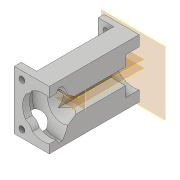
# Autodesk Inventor part: 30_CUBE_OpenSIM_Beamexpander
Saved by Autodesk Inventor 2019 (Build 230136000, 136)
## iProperties
Created: 2019-10-21
Part Number: 30_CUBE_OpenSIM_Beamexpander
Material: Generic
Document SubType Name: Modeling
Designer: diederichbenedict
Density: 1 g/cm^3
Appearance: Default
Author: diederichbenedict
Autodesk Inventor part; units mm, degrees
ref_plane "YZ Plane" through (0, 0, 0) normal (1, 0, 0) x (0, 1, 0)
ref_plane "XZ Plane" through (0, 0, 0) normal (0, 1, 0) x (-1, 0, 0)
ref_plane "XY Plane" through (0, 0, 0) normal (0, 0, 1) x (1, 0, 0)
ref_plane "Work Plane1" through (0, 0, 0) normal (0, 0, 1) x (1, 0, 0)
sketch "Sketch1" plane through (0, 0, 0) normal (0, 0, 1) x (1, 0, 0)
  circle A0 centre (11, -11) radius 1 projected
  circle A1 centre (-11, -11) radius 1 projected
  circle A2 centre (-11, 11) radius 1 projected
  circle A3 centre (11, 11) radius 1 projected
  circle A4 centre (0, 0) radius 2.8472 projected
  circle A5 centre (0, 0) radius 9.9557 construction
  line L0 (12.95, 14.95) -> (-12.95, 14.95) construction
  arc A6 (-12.95, 14.95) -> (-14.95, 12.95) centre (-12.95, 12.95) ccw construction
  line L1 (-14.95, 12.95) -> (-14.95, -12.95) construction
  arc A7 (-14.95, -12.95) -> (-12.95, -14.95) centre (-12.95, -12.95) ccw construction
  line L2 (-12.95, -14.95) -> (12.95, -14.95) construction
  arc A8 (12.95, -14.95) -> (14.95, -12.95) centre (12.95, -12.95) ccw construction
  line L3 (14.95, -12.95) -> (14.95, 12.95) construction
  arc A9 (14.95, 12.95) -> (12.95, 14.95) centre (12.95, 12.95) ccw construction
  line L4 (-14.95, -14.95) -> (10.05, -14.95) construction
  line L5 (10.05, -14.95) -> (10.05, 14.95) construction
  line L6 (10.05, 14.95) -> (-14.95, 14.95) construction
  line L7 (-14.95, 14.95) -> (-14.95, -14.95) construction
  line L8 (-14.95, -14.95) -> (10.05, -14.95)
  line L9 (10.05, -14.95) -> (10.05, 14.95)
  line L10 (10.05, 14.95) -> (-14.95, 14.95)
  line L11 (-14.95, 14.95) -> (-14.95, -14.95)
  circle A10 centre (-11, -11) radius 1.5
  circle A11 centre (-11, 11) radius 1.5
  line L12 (2.9776, -9.5) -> (2.9776, -14.95)
  line L13 (2.9776, 9.5) -> (2.9776, 14.95)
  arc A12 (2.9776, 9.5) -> (2.9776, -9.5) centre (0, 0) ccw
  point P0 (0, 0)
  dimension "d0" = 25
  dimension "d1" = 3
  dimension "d2" = 3
  constraints: 20 end point, 5 point on line, 4 parallel, 4 point on circle, 3 centre point, 3 perpendicular, 2 coincident, 2 horizontal, 1 concentric
  measures "d0" distance of L6.end L5.end
  measures "d1" diameter of A10
  measures "d2" diameter of A11
extrude "Extrusion1" add sketch "Sketch1" along normal blind 3 contours L8 L11 L10 L13 A12 L12
sketch "Sketch2" plane through (0, 0, 3) normal (0, 0, 1) x (1, 0, 0)
  circle A0 centre (-11, 11) radius 1.5 projected
  circle A1 centre (-11, -11) radius 1.5 projected
  line L0 (-14.95, -14.95) -> (2.9776, -14.95) projected
  line L1 (2.9776, -14.95) -> (2.9776, -9.5) projected
  arc A2 (2.9776, 9.5) -> (2.9776, -9.5) centre (0, 0) ccw projected
  line L2 (2.9776, 9.5) -> (2.9776, 14.95) projected
  line L3 (2.9776, 14.95) -> (-14.95, 14.95) projected
  line L4 (-14.95, 14.95) -> (-14.95, -14.95) projected
  line L5 (2.9776, -9.5) -> (2.9776, 9.5)
  circle A3 centre (-11, -11) radius 1.5 projected
  line L6 (-14.95, -14.95) -> (2.9776, -14.95) projected
  circle A4 centre (-11, -11) radius 5.5861
  line L7 (2.9776, 14.95) -> (-14.95, 14.95) projected
  circle A5 centre (-11, 11) radius 5.5861
  arc A6 (2.9776, 9.5) -> (2.9776, -9.5) centre (0, 0) ccw projected
  circle A7 centre (0, 0) radius 2.9776
  line L8 (0, -2.9776) -> (2.9776, -2.9776)
  line L9 (0, 2.9776) -> (2.9776, 2.9776)
  point P0 (0, 0)
  point P1 (-14.95, -7.05)
  point P2 (-7.0295, -7.05)
  point P3 (-7.05, -14.95)
  point P4 (-7.05, 7.05)
  point P5 (-14.95, 7.05)
  point P6 (-7.05, 14.95)
  constraints: 10 point on circle, 6 end point, 6 point on line, 3 centre point, 3 coincident, 2 perpendicular, 1 tangent, 1 vertical
extrude "Extrusion2" add sketch "Sketch2" along normal blind 3 contours A4 L4 A5 L3 L2 A2 L1 L0 | A2 L5 L9 A7 L8
sketch "Sketch3" plane through (0, 0, 6) normal (0, 0, 1) x (1, 0, 0)
  line L0 (-4.1, -3.85) -> (-4.1, 3.85) construction
  line L1 (4.1, -3.85) -> (-4.1, -3.85) construction
  line L2 (-4.1, 3.85) -> (4.1, 3.85) construction
  line L3 (4.1, 3.85) -> (4.1, -3.85) construction
  line L4 (4.4, 4.15) -> (-4.4, 4.15)
  line L5 (-4.4, 4.15) -> (-4.4, -4.15)
  line L6 (-4.4, -4.15) -> (4.4, -4.15)
  line L7 (4.4, -4.15) -> (4.4, 4.15)
  line L8 (2.9776, -14.95) -> (2.9776, -2.9776) projected
  line L9 (2.9776, -2.9776) -> (0, -2.9776) projected
  arc A0 (0, 2.9776) -> (0, -2.9776) centre (0, 0) ccw projected
  line L10 (0, 2.9776) -> (2.9776, 2.9776) projected
  line L11 (2.9776, 2.9776) -> (2.9776, 14.95) projected
  line L12 (2.9776, 14.95) -> (-7.05, 14.95) projected
  arc A1 (-14.95, 7.05) -> (-7.05, 14.95) centre (-11, 11) ccw projected
  line L13 (-14.95, 7.05) -> (-14.95, -7.05) projected
  arc A2 (-7.05, -14.95) -> (-14.95, -7.05) centre (-11, -11) ccw projected
  line L14 (-7.05, -14.95) -> (2.9776, -14.95) projected
  line L15 (2.9776, -14.95) -> (2.9776, -2.9776) projected
  point P0 (0, 0)
  point P1 (-13.95, 5)
  point P2 (2.9776, 4.15)
  point P3 (2.9776, -4.15)
  dimension "d7" = 0.3
  constraints: 8 end point, 4 point on line, 4 other
  measures "d7" distance between parallel lines of L2 L4
extrude "Extrusion3" add sketch "Sketch3" along normal blind 5 contours L4 L5 L6 L8 L14 A2 L13 A1 L12 L11
sketch "Sketch4" plane through (0, 0, 11) normal (0, 0, 1) x (1, 0, 0)
  line L0 (-4.4, 4.15) -> (2.9776, 4.15) projected
  line L1 (2.9776, 4.15) -> (2.9776, 14.95) projected
  line L2 (2.9776, 14.95) -> (-7.05, 14.95) projected
  arc A0 (-14.95, 7.05) -> (-7.05, 14.95) centre (-11, 11) ccw projected
  line L3 (-14.95, 7.05) -> (-14.95, -7.05) projected
  arc A1 (-7.05, -14.95) -> (-14.95, -7.05) centre (-11, -11) ccw projected
  line L4 (-7.05, -14.95) -> (2.9776, -14.95) projected
  line L5 (2.9776, -14.95) -> (2.9776, -4.15) projected
  line L6 (2.9776, -4.15) -> (-4.4, -4.15) projected
  line L7 (-4.4, -4.15) -> (-4.4, 4.15) projected
  point P0 (0, 0)
extrude "Extrusion4" add sketch "Sketch4" along normal blind 35
ref_plane "Work Plane2" through (0, 0, 28) normal (0, 0, 1) x (1, 0, 0)
sketch "Sketch5" plane through (0, 0, 28) normal (0, 0, 1) x (1, 0, 0)
  point P0 (0, 0)
ref_plane "Work Plane4" through (-4.4, -0.2931, 6) normal (0, 1, 0) x (1, 0, 0)
ref_plane "Work Plane3" through (2.9776, 3.5638, 6) normal (0, 1, 0) x (1, 0, 0)
sketch "Sketch6" plane through (-4.4, -0.2931, 6) normal (0, 1, 0) x (1, 0, 0)
  line L0 (4.4, -27.526) -> (4.4, 207.156)
  line L1 (4.4, -35.2902) -> (-8.1, -35.2902)
  line L2 (-8.1, -35.2902) -> (-8.1, -33.2902)
  line L3 (-8.1, -33.2902) -> (4.4, -33.2902)
  line L4 (4.4, -33.2902) -> (4.4, -35.2902)
  arc A0 (-8.1, -35.2902) -> (4.4, -39.2902) centre (4.4, -17.7589) ccw
  arc A1 (4.4, -29.2902) -> (-8.1, -33.2902) centre (4.4, -50.8214) ccw
  line L5 (7.3776, -40) -> (0, -40) projected
  line L6 (-6.2938, -36.4468) -> (-6.2938, -40)
  line L7 (-1.0139, -40) -> (-10.55, -40) projected
  line L8 (4.4, -40) -> (-6.2938, -40)
  line L9 (4.4, -29.2902) -> (4.4, -17.7589)
  line L10 (4.4, -17.7589) -> (-2.8665, -30.5534)
  line L11 (4.4, -27.526) -> (4.4, -29.2902)
  line L12 (4.4, -39.2902) -> (4.4, -40)
  line L13 (4.4, -39.2902) -> (4.4, -35.2902)
  line L14 (4.4, -33.2902) -> (4.4, -29.2902)
  point P0 (4.4, 6)
  point P1 (-2.65, -40)
  dimension "d13" = 12.5
  dimension "d14" = 2
  dimension "d15" = 4
  dimension "d16" = 4
  constraints: 24 end point, 6 point on circle, 5 vertical, 2 centre point, 2 parallel, 2 perpendicular, 2 point on line, 1 collinear, 1 horizontal, 11 other
  measures "d13" distance of L3.end L2.end
  measures "d14" distance between parallel lines of L3 L1
  measures "d15" distance from line of L1 L12.start
  measures "d16" distance of L3.end L9.start
revolve "Revolution1" cut sketch "Sketch6" angle 360 about axis through (0, -0.2931, 33.526) along (0, 0, -1)
sketch "Sketch7" plane through (0, 0, 46) normal (0, 0, 1) x (1, 0, 0)
  arc A0 (-7.05, -14.95) -> (-5.6576, -9.3678) centre (-11, -11) ccw projected
  line L0 (-7.05, -14.95) -> (2.9776, -14.95) projected
  line L1 (2.9776, -14.95) -> (2.9776, -10.5641) projected
  line L2 (2.9776, 9.9778) -> (2.9776, 14.95) projected
  line L3 (2.9776, 14.95) -> (-7.05, 14.95) projected
  arc A1 (-5.9636, 8.5835) -> (-7.05, 14.95) centre (-11, 11) ccw projected
  line L4 (-14.95, 7.05) -> (-14.95, -7.05) projected
  arc A2 (-9.2241, -5.7037) -> (-14.95, -7.05) centre (-11, -11) ccw projected
  arc A3 (-7.05, -14.95) -> (-14.95, -7.05) centre (-11, -11) ccw
  arc A4 (-14.95, 7.05) -> (-7.05, 14.95) centre (-11, 11) ccw
  line L5 (-7.05, -14.95) -> (2.9776, -14.95) projected
  line L6 (-7.05, -14.95) -> (-14.95, -14.95)
  line L7 (-14.95, -7.05) -> (-14.95, -14.95)
  line L8 (-14.95, 14.95) -> (-14.95, 7.05) projected
  line L9 (-14.95, 7.05) -> (-14.95, 14.95)
  line L10 (-14.95, 14.95) -> (-7.05, 14.95)
  line L11 (-7.05, -14.95) -> (2.9776, -14.95) projected
  line L12 (2.9776, -14.95) -> (2.9776, -10.5641) projected
  line L13 (2.9776, 9.9778) -> (2.9776, 14.95) projected
  line L14 (2.9776, 14.95) -> (-7.05, 14.95) projected
  arc A5 (-5.9636, 8.5835) -> (-7.05, 14.95) centre (-11, 11) ccw projected
  line L15 (-14.95, 7.05) -> (-14.95, -7.05) projected
  arc A6 (2.9776, 9.9778) -> (-5.9636, 8.5835) centre (0, -0.2931) ccw projected
  arc A7 (-5.6576, -9.3678) -> (2.9776, -10.5641) centre (0, -0.2931) ccw projected
  arc A8 (-7.05, -14.95) -> (-5.6576, -9.3678) centre (-11, -11) ccw projected
  arc A9 (2.9776, 9.9778) -> (-5.9636, 8.5835) centre (0, -0.2931) ccw projected
  arc A10 (-9.2241, -5.7037) -> (-14.95, -7.05) centre (-11, -11) ccw projected
  arc A11 (-5.6576, -9.3678) -> (2.9776, -10.5641) centre (0, -0.2931) ccw projected
  arc A12 (-8.7167, 5.9018) -> (-9.2241, -5.7037) centre (0, -0.2931) ccw projected
  arc A13 (-14.95, 7.05) -> (-8.7167, 5.9018) centre (-11, 11) ccw projected
  arc A14 (-8.7167, 5.9018) -> (-9.2241, -5.7037) centre (0, -0.2931) ccw projected
  arc A15 (-14.95, 7.05) -> (-8.7167, 5.9018) centre (-11, 11) ccw projected
  point P0 (0, 0)
  constraints: 9 end point, 4 point on circle, 2 centre point, 2 coincident, 2 collinear, 2 perpendicular, 2 point on line, 1 concentric
extrude "Extrusion5" add sketch "Sketch7" against normal up to surface (3.5532 mm away) contours L6 L7 A2 A3 A0 | A4 L8 L10 A1
sketch "Sketch8" plane through (0, 0, 46) normal (0, 0, 1) x (1, 0, 0)
  circle A0 centre (-11, -11) radius 1.5 projected
  circle A1 centre (-11, 11) radius 1.5 projected
  point P0 (0, 0)
extrude "Extrusion6" cut sketch "Sketch8" against normal blind 20
sketch "Sketch9" plane through (0, 0, 3) normal (0, 0, -1) x (-1, 0, 0)
  circle A0 centre (0, 0) radius 0.5 projected
  circle A1 centre (0, 0) radius 6.35 projected
  circle A2 centre (0, 0) radius 9.9557
  point P0 (0, 0)
  point P1 (-2.9776, 9.5)
  constraints: 3 other
extrude "Extrusion7" cut sketch "Sketch9" against normal blind 4 contours A1 | A2
sketch "Sketch10" plane through (0, 0, 6) normal (0, 0, 1) x (1, 0, 0)
  line L0 (-4.4, -4.15) -> (2.9776, -4.15) projected
  line L1 (2.9776, -4.15) -> (2.9776, -2.9776) projected
  line L2 (2.9776, -2.9776) -> (0, -2.9776) projected
  arc A0 (0, 2.9776) -> (0, -2.9776) centre (0, 0) ccw projected
  line L3 (0, 2.9776) -> (2.9776, 2.9776) projected
  line L4 (2.9776, 2.9776) -> (2.9776, 4.15) projected
  line L5 (2.9776, 4.15) -> (-4.4, 4.15) projected
  line L6 (-4.4, 4.15) -> (-4.4, -4.15) projected
  point P0 (0, 0)
extrude "Extrusion8" cut sketch "Sketch10" against normal blind 2
body "Solid1"
